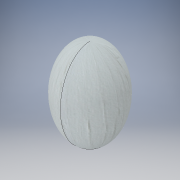
# Autodesk Inventor part: Egg
Saved by Autodesk Inventor 2017 (Build 210142000, 142)
## iProperties
Created: 2017-04-08
Part Number: Egg
Material: Generic
Document SubType Name: Modeling
Designer: Alex Tacescu
Density: 1 g/cm^3
Appearance: Wood - Painted White
Author: Alex Tacescu
Autodesk Inventor part; units mm, degrees
ref_plane "YZ Plane" through (0, 0, 0) normal (1, 0, 0) x (0, 1, 0)
ref_plane "XZ Plane" through (0, 0, 0) normal (0, 1, 0) x (-1, 0, 0)
ref_plane "XY Plane" through (0, 0, 0) normal (0, 0, 1) x (1, 0, 0)
sketch "Sketch1" plane through (0, 0, 0) normal (1, 0, 0) x (0, 1, 0)
  line L0 (0, 0) -> (0, -22.225)
  line L1 (0, 0) -> (33.3595, 0)
  ellipse E0 centre (0, 0) end of major axis (33.3595, 0) minor radius 22.225
  line L2 (-30.1405, 9.525) -> (-30.1405, -9.525)
  line L3 (0, 0) -> (-30.1405, 0)
  line L4 (33.3595, 0) -> (-30.1405, 0)
  dimension "d1" = 22.225
  dimension "d2" = 63.5
  dimension "d3" = 19.05
  constraints: 10 end point, 3 horizontal, 2 vertical, 1 coincident, 1 midpoint, 1 perpendicular, 6 other
  measures "d1" distance of L0.start L0.end
  measures "d2" distance from line of L2 L1.end
  measures "d3" distance of L2.start L2.end
revolve "Revolution1" add sketch "Sketch1" angle 360 about axis through (0, 0, 0) along (0, -1, 0) contours L3 L2 E0 L1
body "Solid1"
